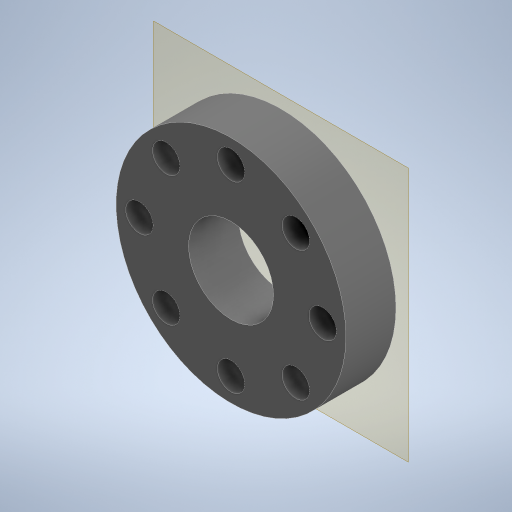
# Autodesk Inventor part: 25
Saved by Autodesk Inventor 2024.3 (Build 283343000, 343)
## iProperties
Created: 2024-09-07
Part Number: 25
Material: 아크릴, 선명
Document SubType Name: Modeling
Designer: 구지현
Density: 1.19 g/cm^3
Appearance: 회색
Author: 구지현
Autodesk Inventor part; units mm, degrees
ref_plane "YZ Plane" through (0, 0, 0) normal (1, 0, 0) x (0, 1, 0)
ref_plane "XZ Plane" through (0, 0, 0) normal (0, 1, 0) x (-1, 0, 0)
ref_plane "XY Plane" through (0, 0, 0) normal (0, 0, 1) x (1, 0, 0)
ref_plane "작업 평면1" through (0, 0, 0) normal (0, 0, 1) x (1, 0, 0)
sketch "스케치1" plane through (0, 0, 0) normal (0, 0, 1) x (1, 0, 0)
  circle A0 centre (-7.778175, -7.778175) radius 1.55
  circle A1 centre (7.778175, -7.778175) radius 1.55
  circle A2 centre (7.778175, 7.778175) radius 1.55
  circle A3 centre (-7.778175, 7.778175) radius 1.55
  circle A4 centre (0, 0) radius 5
  circle A5 centre (0, 0) radius 13.9
  circle A6 centre (0, 11) radius 1.55
  circle A7 centre (11, 0) radius 1.55
  circle A8 centre (0, -11) radius 1.55
  circle A9 centre (-11, 0) radius 1.55
  circle A10 centre (-11, 0) radius 1.65
  circle A11 centre (-7.778175, 7.778175) radius 1.65
  circle A12 centre (0, 11) radius 1.65
  circle A13 centre (7.778175, 7.778175) radius 1.65
  circle A14 centre (11, 0) radius 1.65
  circle A15 centre (7.778175, -7.778175) radius 1.65
  circle A16 centre (0, -11) radius 1.65
  circle A17 centre (-7.778175, -7.778175) radius 1.65
  circle A18 centre (0, 0) radius 5.1
  circle A19 centre (0, 0) radius 13.8
  point P0 (0, 0)
  dimension "d0" = 0.1
  dimension "d1" = 0.1
  dimension "d2" = 0.1
  dimension "d3" = 0.1
  dimension "d4" = 0.1
  dimension "d5" = 0.1
  dimension "d6" = 0.1
  dimension "d7" = 0.1
  dimension "d8" = 0.1
  dimension "d9" = 0.1
  constraints: 10 centre point
  measures "d0" radial gap between concentric circles of A9 A10
  measures "d1" radial gap between concentric circles of A3 A11
  measures "d2" radial gap between concentric circles of A6 A12
  measures "d3" radial gap between concentric circles of A2 A13
  measures "d4" radial gap between concentric circles of A7 A14
  measures "d5" radial gap between concentric circles of A1 A15
  measures "d6" radial gap between concentric circles of A8 A16
  measures "d7" radial gap between concentric circles of A0 A17
  measures "d8" radial gap between concentric circles of A4 A18
  measures "d9" radial gap between concentric circles of A5 A19
sketch "스케치1 outline for 돌출1" plane through (0, 0, 0) normal (0, 0, 1) x (1, 0, 0)
  circle A0 centre (0, 0) radius 13.8
  circle A1 centre (-7.778175, -7.778175) radius 1.65
  circle A2 centre (-11, 0) radius 1.65
  circle A3 centre (0, -11) radius 1.65
  circle A4 centre (7.778175, -7.778175) radius 1.65
  circle A5 centre (0, 0) radius 5.1
  circle A6 centre (11, 0) radius 1.65
  circle A7 centre (-7.778175, 7.778175) radius 1.65
  circle A8 centre (0, 11) radius 1.65
  circle A9 centre (7.778175, 7.778175) radius 1.65
extrude "돌출1" add sketch "스케치1 outline for 돌출1" along normal blind 6
